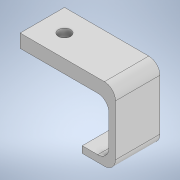
# Autodesk Inventor part: Cable_Guide_Holder
Saved by Autodesk Inventor 2021 (Build 250183000, 183)
## iProperties
Created: 2021-08-21
Part Number: Cable_Guide_Holder
Material: Generic
Document SubType Name: Modeling
Designer: Jorian Bruslind
Density: 1 g/cm^3
Appearance: Default
Author: Jorian Bruslind
Autodesk Inventor part; units mm, degrees
ref_plane "YZ Plane" through (0, 0, 0) normal (1, 0, 0) x (0, 1, 0)
ref_plane "XZ Plane" through (0, 0, 0) normal (0, 1, 0) x (-1, 0, 0)
ref_plane "XY Plane" through (0, 0, 0) normal (0, 0, 1) x (1, 0, 0)
sketch "Sketch1" plane through (0, 0, 0) normal (0, 1, 0) x (-1, 0, 0)
  line L0 (0, 0) -> (40, 0)
  line L1 (40, 0) -> (40, -20)
  line L2 (40, -20) -> (0, -20)
  line L3 (0, -20) -> (0, 0)
  dimension "d0" = 40
  dimension "d1" = 20
  constraints: 8 end point, 2 parallel, 1 horizontal, 1 perpendicular
  measures "d0" distance of L1.end L2.end
  measures "d1" distance of L0.end L1.end
extrude "Extrusion1" add sketch "Sketch1" along normal blind 6
sketch "Sketch2" plane through (0, 6, 0) normal (0, 1, 0) x (1, 0, 0)
  line L0 (0, 0) -> (3, 0)
  line L1 (3, 0) -> (3, 20)
  line L2 (3, 20) -> (0, 20)
  line L3 (0, 20) -> (0, 0)
  dimension "d4" = 3
  dimension "d5" = 20
  constraints: 8 end point, 2 parallel, 1 horizontal, 1 perpendicular
  measures "d4" distance of L2.end L1.end
  measures "d5" distance of L1.end L0.end
extrude "Extrusion2" add sketch "Sketch2" against normal blind 30
fillet "Fillet1" radius 5 1 edges at (0, 0, -10)
fillet "Fillet4" radius 5 1 edges at (3, 6, -10)
sketch "Sketch5" plane through (0, 0, 0) normal (0, -1, 0) x (1, 0, 0)
  circle A0 centre (-30, -10) radius 2.75
  line L0 (-40, -20) -> (-40, 0) projected
  line L1 (-5, -20) -> (-40, -20) projected
  point P0 (0, 0)
  dimension "d18" = 5.5
  dimension "d19" = 10
  dimension "d20" = 10
  constraints: 1 centre point
  measures "d18" diameter of A0
  measures "d19" distance from line of L0 A0.centre
  measures "d20" distance from line of L1 A0.centre
extrude "Extrusion4" cut sketch "Sketch5" against normal through all
sketch "Sketch7" plane through (3, -24, 0) normal (1, 0, 0) x (0, 0, -1)
  line L0 (0, 0) -> (20, 0) projected
  line L1 (0, 0) -> (20, 0)
  line L2 (20, 0) -> (20, -3)
  line L3 (20, -3) -> (0, -3)
  line L4 (0, -3) -> (0, 0)
  point P0 (0, 24)
  dimension "d26" = 20
  dimension "d27" = 3
  constraints: 8 end point, 2 parallel, 1 horizontal, 1 perpendicular
  measures "d26" distance of L2.end L3.end
  measures "d27" distance of L1.end L2.end
extrude "Extrusion5" add sketch "Sketch7" against normal blind 15
fillet "Fillet6" radius 5 2 edges at (0, -24, -10) (3, -27, -10)
body "Solid1"
